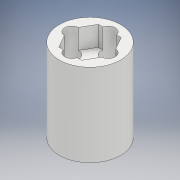
# Autodesk Inventor part: AA032
Saved by Autodesk Inventor 2017 SP1 (Build 210196100, 196)
## iProperties
Created: 2017-10-13
Part Number: AA032
Material: ABS Plastic
Document SubType Name: Modeling
Designer: Zach
Density: 1.06 g/cm^3
Appearance: CR White
Author: Zach
Autodesk Inventor part; units mm, degrees
ref_plane "YZ Plane" through (0, 0, 0) normal (1, 0, 0) x (0, 1, 0)
ref_plane "XZ Plane" through (0, 0, 0) normal (0, 1, 0) x (-1, 0, 0)
ref_plane "XY Plane" through (0, 0, 0) normal (0, 0, 1) x (1, 0, 0)
sketch "Sketch1" plane through (0, 0, 0) normal (0, 0, 1) x (1, 0, 0)
  circle A0 centre (0, 0) radius 10.75
  circle A1 centre (0, 0) radius 2.25
  dimension "d0" = 21.5
  dimension "d1" = 4.5
  constraints: 2 centre point, 2 coincident
  measures "d0" diameter of A0
  measures "d1" diameter of A1
extrude "Extrusion1" add sketch "Sketch1" along normal blind 29
sketch "Sketch2" plane through (0, 0, 29) normal (0, 0, 1) x (1, 0, 0)
  line L0 (8, 0) -> (4, -6.9282)
  line L1 (4, -6.9282) -> (-4, -6.9282)
  line L2 (-4, -6.9282) -> (-8, 0)
  line L3 (-8, 0) -> (-4, 6.9282)
  line L4 (-4, 6.9282) -> (4, 6.9282)
  line L5 (4, 6.9282) -> (8, 0)
  point P0 (0, 0)
  point P1 (0, 0)
  dimension "d4" = 16
  constraints: 12 end point, 1 coincident, 1 horizontal alignment, 13 other
  measures "d4" distance of L0.start L2.end
extrude "Extrusion2" cut sketch "Sketch2" against normal blind 7
sketch "Sketch9" plane through (0, 0, 29) normal (0, 0, 1) x (1, 0, 0)
  circle A0 centre (0, -6.35) radius 1.5
  circle A1 centre (0, 6.35) radius 1.5
  line L0 (0, 6.35) -> (0, -6.35) construction
  circle A2 centre (6.35, 0) radius 1.5
  circle A3 centre (-6.35, 0) radius 1.5
  line L1 (-6.35, 0) -> (6.35, 0) construction
  point P0 (0, 0)
  point P1 (0, 0)
  dimension "d19" = 3
  dimension "d20" = 3
  dimension "d21" = 12.7
  dimension "d22" = 3
  dimension "d23" = 3
  dimension "d24" = 12.7
  constraints: 4 centre point, 4 end point, 2 coincident, 2 midpoint, 1 horizontal, 1 vertical
  measures "d19" diameter of A0
  measures "d20" diameter of A1
  measures "d21" distance of L0.start L0.end
  measures "d22" diameter of A2
  measures "d23" diameter of A3
  measures "d24" distance of L1.start L1.end
extrude "Extrusion6" cut sketch "Sketch9" against normal through all
ref_plane "Work Plane2" through (0, 0, 5) normal (0, 0, -1) x (-1, 0, 0)
sketch "Sketch11" plane through (0, 0, 5) normal (0, 0, -1) x (-1, 0, 0)
  circle A0 centre (-6.35, 0) radius 1.5 projected
  spline S0 degree 2 poles (-1.5, 6.35) (-1.5, 8.9481) (0.75, 7.649) (3, 6.35) (0.75, 5.051) (-1.5, 3.7519) (-1.5, 6.35) knots 0 0 0 0.333333 0.333333 0.666667 0.666667 1 1 1 weights 1 0.5 1 0.5 1 0.5 1 projected
  circle A1 centre (6.35, 0) radius 1.5 projected
  circle A2 centre (-6.35, 0) radius 2.5
  circle A3 centre (0, 6.35) radius 1.5 projected
  circle A4 centre (0, 6.35) radius 2.5
  circle A5 centre (6.35, 0) radius 2.5
  circle A6 centre (0, -6.35) radius 1.5 projected
  circle A7 centre (0, -6.35) radius 2.5
  point P0 (0, 0)
  dimension "d32" = 5
  dimension "d33" = 5
  dimension "d34" = 5
  dimension "d35" = 5
  constraints: 4 centre point, 4 coincident, 1 horizontal alignment, 1 other
  measures "d32" diameter of A2
  measures "d33" diameter of A4
  measures "d34" diameter of A5
  measures "d35" diameter of A7
extrude "Extrusion7" cut sketch "Sketch11" against normal through all contours A0 | S0 | A1 | A2 | A4 | A5 | A6 | A7
body "Solid1"
